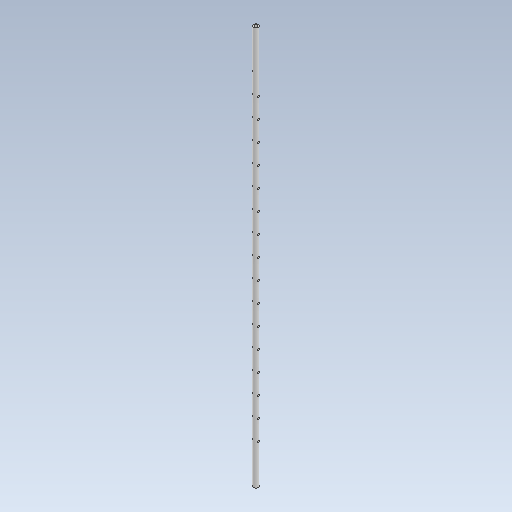
# Autodesk Inventor part: burder_rod_2
Saved by Autodesk Inventor 2020 (Build 240168000, 168)
## iProperties
Created: 2019-06-12
Part Number: burder_rod_2
Material: Generic
Document SubType Name: Modeling
Designer: ColinP
Density: 1 g/cm^3
Appearance: Default
Mass: 1.26312 g
Surface Area: 40.7053 cm^2
Volume: 1.26312 cm^3
Author: ColinP
Autodesk Inventor part; units mm, degrees
ref_plane "YZ Plane" through (0, 0, 0) normal (1, 0, 0) x (0, 1, 0)
ref_plane "XZ Plane" through (0, 0, 0) normal (0, 1, 0) x (-1, 0, 0)
ref_plane "XY Plane" through (0, 0, 0) normal (0, 0, 1) x (1, 0, 0)
sketch "Sketch1" plane through (0, 0, 0) normal (0, 1, 0) x (-1, 0, 0)
  circle A0 centre (0, 0) radius 1.5875
  dimension "d0" = 3.175
  constraints: 1 centre point, 1 coincident
  measures "d0" diameter of A0
extrude "Extrusion1" add sketch "Sketch1" along normal blind 254
sketch "Sketch9" plane through (0, 0, 0) normal (1, 0, 0) x (0, 1, 0)
  line L0 (0, -1.5875) -> (0, 1.5875) projected
  line L1 (254, -1.5875) -> (254, 1.5875) projected
  line L2 (254, 0) -> (228.6, 0)
  line L3 (0, 0) -> (25.4, 0)
  dimension "d42" = 25.4
  dimension "d43" = 25.4
  constraints: 4 end point, 2 horizontal, 1 midpoint
  measures "d42" distance of L2.start L2.end
  measures "d43" distance of L3.start L3.end
hole "Hole5" at (0, 25.4, 0) direction (-1, 0, 0) diameter 1.1906 end through all both
hole "Hole6" at (0, 228.6, 0) direction (-1, 0, 0) diameter 1.27 end through all
sketch "Sketch10" plane through (0, 254, 0) normal (0, 1, 0) x (1, 0, 0)
  circle A0 centre (0, 0) radius 1.5875 projected
  constraints: 1 coincident
hole "Hole7" at (0, 254, 0) direction (0, -1, 0) diameter 1.905 end through all
sketch "Sketch11" plane through (0, 0, 0) normal (1, 0, 0) x (0, 1, 0)
  line L0 (0, 0) -> (25.4, 0)
  line L1 (25.4, 0) -> (50.8, 0)
  dimension "d65" = 25.4
  dimension "d66" = 25.4
  dimension "d67" = 180
  constraints: 4 end point, 1 collinear, 1 horizontal
  measures "d65" distance of L0.start L0.end
  measures "d66" distance of L0.end L1.end
  measures "d67" angle of L1 L0
pattern_linear "Rectangular Pattern1" count 16 spacing 12.7 along (0, 1, 0) of "Hole5"
body "Solid1"
